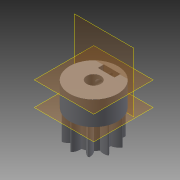
# Autodesk Inventor part: sj-small-gear
Saved by Autodesk Inventor 2014 (Build 180170000, 170)
## iProperties
Created: 2013-11-16
Part Number: sj-small-gear
Material: Generic
Document SubType Name: Modeling
Designer: stephen
Density: 1 g/cm^3
Appearance: Default
Author: stephen
Autodesk Inventor part; units mm, degrees
ref_plane "YZ Plane" through (0, 0, 0) normal (1, 0, 0) x (0, 1, 0)
ref_plane "XZ Plane" through (0, 0, 0) normal (0, 1, 0) x (-1, 0, 0)
ref_plane "XY Plane" through (0, 0, 0) normal (0, 0, 1) x (1, 0, 0)
ref_plane "Work Plane1" through (0, 0, 8) normal (0, 0, 1) x (1, 0, 0)
sketch "Sketch1" plane through (0, 0, 0) normal (0, 0, 1) x (1, 0, 0)
  circle A0 centre (0, 0) radius 2.6023
  line L0 (-0.1767, 8.453) -> (0.1689, 8.453)
  line L1 (0.1689, 8.453) -> (0.9579, 5.5085) construction
  arc A1 (-0.1767, 8.453) -> (-0.9656, 5.5084) centre (2.8217, 6.0717) ccw
  line L2 (-5.1115, 6.7348) -> (-4.8319, 6.9379)
  arc A2 (-2.4629, 5.0195) -> (-4.8319, 6.9379) centre (-5.8579, 3.249) ccw
  line L3 (-4.8319, 6.9379) -> (-2.4629, 5.0195) construction
  arc A3 (-5.1115, 6.7348) -> (-4.0189, 3.8888) centre (-1.286, 6.5706) ccw
  line L4 (-8.0939, 2.4441) -> (-7.9871, 2.7727)
  arc A4 (-4.9429, 2.6132) -> (-7.9871, 2.7727) centre (-6.6488, -0.8147) ccw
  line L5 (-7.9871, 2.7727) -> (-4.9429, 2.6132) construction
  arc A5 (-8.0939, 2.4441) -> (-5.5371, 0.7838) centre (-4.9025, 4.5598) ccw
  line L6 (-7.9847, -2.7801) -> (-8.0915, -2.4515)
  arc A6 (-5.5349, -0.7913) -> (-8.0915, -2.4515) centre (-4.9001, -4.5672) ccw
  line L7 (-8.0915, -2.4515) -> (-5.5349, -0.7913) construction
  arc A7 (-7.9847, -2.7801) -> (-4.9404, -2.6205) centre (-6.6464, 0.8073) ccw
  line L8 (-4.8256, -6.9425) -> (-5.1052, -6.7393)
  arc A8 (-4.0128, -3.8935) -> (-5.1052, -6.7393) centre (-1.2798, -6.5752) ccw
  line L9 (-5.1052, -6.7393) -> (-4.0128, -3.8935) construction
  line L10 (0.1767, -8.453) -> (-0.1689, -8.453)
  arc A9 (-0.9579, -5.5085) -> (-0.1689, -8.453) centre (2.8295, -6.0717) ccw
  line L11 (-0.1689, -8.453) -> (-0.9579, -5.5085) construction
  arc A10 (0.1767, -8.453) -> (0.9656, -5.5084) centre (-2.8217, -6.0717) ccw
  line L12 (5.1115, -6.7348) -> (4.8319, -6.9379)
  arc A11 (2.4629, -5.0195) -> (4.8319, -6.9379) centre (5.8579, -3.249) ccw
  line L13 (4.8319, -6.9379) -> (2.4629, -5.0195) construction
  arc A12 (5.1115, -6.7348) -> (4.0189, -3.8888) centre (1.286, -6.5706) ccw
  line L14 (8.0939, -2.4441) -> (7.9871, -2.7727)
  arc A13 (3.3182, -1.074) -> (8.2332, -2.671) centre (6.6488, 0.8147) ccw
  line L15 (7.9871, -2.7727) -> (4.9429, -2.6132) construction
  line L16 (7.9847, 2.7801) -> (8.0915, 2.4515)
  arc A14 (5.5349, 0.7913) -> (8.0915, 2.4515) centre (4.9001, 4.5672) ccw
  line L17 (8.0915, 2.4515) -> (4.0908, -0.1465) construction
  arc A15 (7.9847, 2.7801) -> (4.9404, 2.6205) centre (6.6464, -0.8073) ccw
  line L18 (4.8256, 6.9425) -> (5.1052, 6.7393)
  arc A16 (4.0128, 3.8935) -> (5.1052, 6.7393) centre (1.2798, 6.5752) ccw
  line L19 (5.1052, 6.7393) -> (4.0128, 3.8935) construction
  arc A17 (-5.5371, 0.7838) -> (-5.536, -0.7919) centre (0, 0) ccw
  arc A18 (-4.0189, 3.8888) -> (-4.9442, 2.6133) centre (0, 0) ccw
  arc A19 (2.4565, 5.0239) -> (0.9575, 5.5098) centre (0, 0) ccw
  arc A20 (4.9404, 2.6205) -> (4.0132, 3.8947) centre (0, 0) ccw
  arc A21 (4.9442, -2.6133) -> (5.536, 0.7919) centre (0, 0) ccw
  arc A22 (2.4639, -5.0203) -> (4.9442, -2.6133) centre (0, 0) ccw
  arc A23 (0.9656, -5.5084) -> (2.4639, -5.0203) centre (0, 0) ccw
  arc A24 (-4.9404, -2.6205) -> (-4.0132, -3.8947) centre (0, 0) ccw
  arc A25 (-2.4565, -5.0239) -> (-0.9575, -5.5098) centre (0, 0) ccw
  arc A26 (0.9579, 5.5085) -> (0.1689, 8.453) centre (-2.8295, 6.0717) ccw
  arc A27 (-2.1474, 2.3039) -> (-1.5764, 2.4536) centre (-2.8295, 6.0717) ccw
  arc A28 (-3.1006, 2.2523) -> (-3.0363, 2.2483) centre (-2.8295, 6.0717) ccw
  arc A29 (4.8256, 6.9425) -> (2.4565, 5.0239) centre (5.8516, 3.2535) ccw
  circle A30 centre (4.9025, -4.5598) radius 3.829
  arc A31 (1.7403, -2.4009) -> (1.7114, -2.4439) centre (4.9025, -4.5598) ccw
  arc A32 (1.1846, -3.6447) -> (1.1248, -3.9359) centre (4.9025, -4.5598) ccw
  arc A33 (-4.8256, -6.9425) -> (-2.4565, -5.0239) centre (-5.8516, -3.2535) ccw
  arc A34 (-2.1424, -2.3034) -> (-2.3452, -1.7153) centre (-5.8516, -3.2535) ccw
  arc A35 (-0.9656, 5.5084) -> (-2.4639, 5.0203) centre (0, 0) ccw
  arc A36 (-4.0189, 3.8888) -> (-4.9442, 2.6133) centre (0, 0) ccw
  point P0 (-0.7682, 6.1639)
  point P1 (0.7605, 6.1646)
  point P2 (-4.2445, 4.5351)
  point P3 (-3.0082, 5.4342)
  point P4 (-6.0996, 1.1741)
  point P5 (-5.6279, 2.6282)
  point P6 (-5.6248, -2.6354)
  point P7 (-6.0979, -1.1817)
  point P8 (-3.0015, -5.4382)
  point P9 (-4.2387, -4.5403)
  point P10 (0.7682, -6.1639)
  point P11 (-0.7605, -6.1646)
  point P12 (4.2445, -4.5351)
  point P13 (3.0082, -5.4342)
  point P14 (6.0996, -1.1741)
  point P15 (5.6279, -2.6282)
  point P16 (5.6248, 2.6354)
  point P17 (6.0979, 1.1817)
  point P18 (3.0015, 5.4382)
  point P19 (4.2387, 4.5403)
  constraints: 81 point on circle, 40 end point, 37 centre point, 15 point on line, 4 coincident, 1 horizontal
sketch "Sketch2" plane through (0, 0, 8) normal (0, 0, 1) x (1, 0, 0)
  circle A0 centre (0, 0) radius 2.6023 projected
  arc A1 (-5.2272, 2.3957) -> (-5.6389, 1.125) centre (0, 0) ccw projected
  circle A2 centre (0, 0) radius 8.8963
  dimension "d8" = 17.7926
  constraints: 1 centre point, 1 coincident
  measures "d8" diameter of A2
extrude "Extrusion2" add sketch "Sketch2" along normal blind 8.85
ref_plane "Work Plane2" through (0, 0, 16.85) normal (0, 0, 1) x (1, 0, 0)
sketch "Sketch3" plane through (0, 0, 16.85) normal (0, 0, 1) x (1, 0, 0)
  circle A0 centre (0, 0) radius 2.6023 projected
  circle A1 centre (0, 0) radius 8.8963 projected
  line L0 (0, 6.8373) -> (3.0745, 6.8373)
  line L1 (3.0745, 6.8373) -> (3.0745, 4.6023)
  line L2 (3.0745, 4.6023) -> (0, 4.6023)
  line L3 (0, 6.8373) -> (-3.0745, 6.8373)
  line L4 (-3.0745, 6.8373) -> (-3.0745, 4.6023)
  line L5 (-3.0745, 4.6023) -> (0, 4.6023)
  line L6 (0, -4.8344) -> (3.0745, -4.8344)
  line L7 (3.0745, -4.8344) -> (3.0745, -7.0696)
  line L8 (3.0745, -7.0696) -> (0, -7.0696)
  line L9 (0, -4.8344) -> (-3.0745, -4.8344)
  line L10 (-3.0745, -4.8344) -> (-3.0745, -7.0696)
  line L11 (-3.0745, -7.0696) -> (0, -7.0696)
  line L12 (0, -9.0696) -> (0, -7.0696)
  line L13 (0, 2.6023) -> (0, 3.7788)
  line L14 (0, 3.7788) -> (0, 4.6023)
  dimension "d10" = 2.235
  dimension "d11" = 2
  dimension "d31" = 2.2352
  dimension "d32" = 6.149
  dimension "d33" = 6.149
  constraints: 30 end point, 3 collinear, 3 perpendicular, 2 horizontal, 2 parallel, 1 vertical, 1 vertical alignment, 1 other
  measures "d10" distance of L0.end L1.end
  measures "d31" distance of L6.end L7.end
  measures "d32" distance between parallel lines of L10 L7
  measures "d33" distance between parallel lines of L4 L1
extrude "Extrusion3" cut sketch "Sketch3" against normal blind 8 contours L5 L4 L3 L0 L1 L2
ref_plane "Work Plane3" through (-2.75, 6.6023, 16.85) normal (0, -1, 0) x (1, 0, 0)
sketch "Sketch4" plane through (-2.75, 6.6023, 16.85) normal (0, -1, 0) x (1, 0, 0)
  line L0 (5.5, 0) -> (5.5, -8) projected
  line L1 (2.75, 0.553) -> (2.75, -3.197)
  circle A0 centre (2.75, -2.8775) radius 1.75
  point P0 (2.75, -16.85)
  dimension "d14" = 3.75
  dimension "d15" = 3.5
  constraints: 2 end point, 1 centre point, 1 parallel, 1 point on line
  measures "d14" distance of L1.start L1.end
  measures "d15" diameter of A0
extrude "Extrusion4" cut sketch "Sketch4" along normal mid plane 9
sketch "Sketch5" plane through (0, 0, 8) normal (0, 0, -1) x (-1, 0, 0)
  circle A0 centre (0, 0) radius 2.6023 projected
  circle A1 centre (0, 0) radius 8.8963 projected
  line L0 (-0.1767, 8.453) -> (0.169, 8.453)
  line L1 (0.1689, 8.453) -> (0.9579, 5.5085) construction
  arc A2 (0.9579, 5.5085) -> (0.1689, 8.453) centre (-2.8295, 6.0717) ccw
  circle A3 centre (0, 0) radius 2.6023
  arc A4 (-0.1767, 8.453) -> (-0.9656, 5.5085) centre (2.8217, 6.0717) ccw
  arc A5 (0.9575, 5.5099) -> (0.169, 8.453) centre (-2.8254, 6.0736) ccw
  line L2 (0.1689, 8.453) -> (-0.1767, 8.453)
  arc A6 (-0.1767, 8.453) -> (-0.9656, 5.5085) centre (2.8217, 6.0717) ccw
  line L3 (-5.1115, 6.7348) -> (-4.8318, 6.9379)
  line L4 (-4.8319, 6.9379) -> (-2.4629, 5.0195) construction
  arc A7 (-2.4629, 5.0195) -> (-4.8319, 6.9379) centre (-5.8579, 3.249) ccw
  arc A8 (-5.1115, 6.7348) -> (-4.019, 3.8889) centre (-1.286, 6.5706) ccw
  arc A9 (-2.464, 5.0204) -> (-4.8318, 6.9379) centre (-5.8558, 3.2529) ccw
  line L5 (-4.8319, 6.9379) -> (-5.1115, 6.7348)
  arc A10 (-5.1115, 6.7348) -> (-4.019, 3.8889) centre (-1.286, 6.5706) ccw
  line L6 (-8.0939, 2.4441) -> (-7.987, 2.7728)
  line L7 (-7.9871, 2.7727) -> (-4.9429, 2.6132) construction
  arc A11 (-4.9429, 2.6132) -> (-7.9871, 2.7727) centre (-6.6488, -0.8147) ccw
  arc A12 (-8.0939, 2.4441) -> (-5.5373, 0.7839) centre (-4.9025, 4.5598) ccw
  arc A13 (-4.9444, 2.6133) -> (-7.987, 2.7728) centre (-6.6494, -0.8103) ccw
  line L8 (-7.9871, 2.7727) -> (-8.0939, 2.4441)
  arc A14 (-8.0939, 2.4441) -> (-5.5373, 0.7839) centre (-4.9025, 4.5598) ccw
  line L9 (-7.9847, -2.7801) -> (-8.0915, -2.4514)
  line L10 (-8.0915, -2.4515) -> (-5.5349, -0.7913) construction
  arc A15 (-5.5349, -0.7913) -> (-8.0915, -2.4515) centre (-4.9001, -4.5672) ccw
  arc A16 (-7.9847, -2.7801) -> (-4.9405, -2.6206) centre (-6.6464, 0.8073) ccw
  arc A17 (-5.5361, -0.792) -> (-8.0915, -2.4514) centre (-4.9032, -4.564) ccw
  line L11 (-8.0915, -2.4515) -> (-7.9847, -2.7801)
  arc A18 (-7.9847, -2.7801) -> (-4.9405, -2.6206) centre (-6.6464, 0.8073) ccw
  line L12 (-4.8256, -6.9425) -> (-5.1053, -6.7393)
  line L13 (-5.1052, -6.7393) -> (-4.0128, -3.8935) construction
  arc A19 (-4.0128, -3.8935) -> (-5.1052, -6.7393) centre (-1.2798, -6.5752) ccw
  arc A20 (-4.8256, -6.9425) -> (-2.4566, -5.0241) centre (-5.8516, -3.2535) ccw
  arc A21 (-4.0133, -3.8948) -> (-5.1053, -6.7393) centre (-1.2842, -6.5744) ccw
  line L14 (-5.1052, -6.7393) -> (-4.8256, -6.9425)
  arc A22 (-4.8256, -6.9425) -> (-2.4566, -5.0241) centre (-5.8516, -3.2535) ccw
  line L15 (0.1767, -8.453) -> (-0.169, -8.453)
  line L16 (-0.1689, -8.453) -> (-0.9579, -5.5085) construction
  arc A23 (-0.9579, -5.5085) -> (-0.1689, -8.453) centre (2.8295, -6.0717) ccw
  arc A24 (0.1767, -8.453) -> (0.9656, -5.5085) centre (-2.8217, -6.0717) ccw
  arc A25 (-0.9575, -5.5099) -> (-0.169, -8.453) centre (2.8254, -6.0736) ccw
  line L17 (-0.1689, -8.453) -> (0.1767, -8.453)
  arc A26 (0.1767, -8.453) -> (0.9656, -5.5085) centre (-2.8217, -6.0717) ccw
  line L18 (5.1115, -6.7348) -> (4.8318, -6.9379)
  line L19 (4.8319, -6.9379) -> (2.4629, -5.0195) construction
  arc A27 (2.4629, -5.0195) -> (4.8319, -6.9379) centre (5.8579, -3.249) ccw
  arc A28 (5.1115, -6.7348) -> (4.019, -3.8889) centre (1.286, -6.5706) ccw
  arc A29 (2.464, -5.0204) -> (4.8318, -6.9379) centre (5.8558, -3.2529) ccw
  line L20 (4.8319, -6.9379) -> (5.1115, -6.7348)
  arc A30 (5.1115, -6.7348) -> (4.019, -3.8889) centre (1.286, -6.5706) ccw
  line L21 (8.0939, -2.4441) -> (7.987, -2.7728)
  line L22 (7.9871, -2.7727) -> (4.9429, -2.6132) construction
  arc A31 (4.9429, -2.6132) -> (7.9871, -2.7727) centre (6.6488, 0.8147) ccw
  arc A32 (8.0939, -2.4441) -> (5.5373, -0.7839) centre (4.9025, -4.5598) ccw
  arc A33 (4.9444, -2.6133) -> (7.987, -2.7728) centre (6.6494, 0.8103) ccw
  line L23 (7.9871, -2.7727) -> (8.0939, -2.4441)
  arc A34 (8.0939, -2.4441) -> (5.5373, -0.7839) centre (4.9025, -4.5598) ccw
  line L24 (7.9847, 2.7801) -> (8.0915, 2.4514)
  line L25 (8.0915, 2.4515) -> (5.5349, 0.7913) construction
  arc A35 (5.5349, 0.7913) -> (8.0915, 2.4515) centre (4.9001, 4.5672) ccw
  arc A36 (7.9847, 2.7801) -> (4.9405, 2.6206) centre (6.6464, -0.8073) ccw
  arc A37 (5.5361, 0.792) -> (8.0915, 2.4514) centre (4.9032, 4.564) ccw
  line L26 (8.0915, 2.4515) -> (7.9847, 2.7801)
  arc A38 (7.9847, 2.7801) -> (4.9405, 2.6206) centre (6.6464, -0.8073) ccw
  line L27 (4.8256, 6.9425) -> (5.1053, 6.7393)
  line L28 (5.1052, 6.7393) -> (4.0128, 3.8935) construction
  arc A39 (4.0128, 3.8935) -> (5.1052, 6.7393) centre (1.2798, 6.5752) ccw
  arc A40 (4.8256, 6.9425) -> (2.4566, 5.0241) centre (5.8516, 3.2535) ccw
  arc A41 (4.0133, 3.8948) -> (5.1053, 6.7393) centre (1.2842, 6.5744) ccw
  line L29 (5.1052, 6.7393) -> (4.8256, 6.9425)
  arc A42 (4.8256, 6.9425) -> (2.4566, 5.0241) centre (5.8516, 3.2535) ccw
  arc A43 (2.4566, 5.0241) -> (0.9575, 5.5099) centre (0, 0) ccw
  arc A44 (4.9405, 2.6206) -> (4.0133, 3.8948) centre (0, 0) ccw
  arc A45 (5.5373, -0.7839) -> (5.5361, 0.792) centre (0, 0) ccw
  arc A46 (4.019, -3.8889) -> (4.9444, -2.6133) centre (0, 0) ccw
  arc A47 (0.9656, -5.5085) -> (2.464, -5.0204) centre (0, 0) ccw
  arc A48 (-2.4566, -5.0241) -> (-0.9575, -5.5099) centre (0, 0) ccw
  arc A49 (-4.9405, -2.6206) -> (-4.0133, -3.8948) centre (0, 0) ccw
  arc A50 (-5.5373, 0.7839) -> (-5.5361, -0.792) centre (0, 0) ccw
  arc A51 (-0.9656, 5.5085) -> (-2.464, 5.0204) centre (0, 0) ccw
  arc A52 (-4.019, 3.8889) -> (-4.9444, 2.6133) centre (0, 0) ccw
  point P0 (-0.7682, 6.1639)
  point P1 (0.7605, 6.1646)
  point P2 (-1.286, 6.5706)
  point P3 (1.2798, 6.5752)
  point P4 (0.9575, 5.5098)
  point P5 (-4.9025, 4.5598)
  point P6 (-4.2445, 4.5351)
  point P7 (-2.4639, 5.0203)
  point P8 (-3.0082, 5.4342)
  point P9 (-2.8295, 6.0717)
  point P10 (-6.6464, 0.8073)
  point P11 (-6.0996, 1.1741)
  point P12 (-4.9442, 2.6133)
  point P13 (-5.6279, 2.6282)
  point P14 (-5.8579, 3.249)
  point P15 (-5.8516, -3.2535)
  point P16 (-5.6248, -2.6354)
  point P17 (-5.536, -0.7919)
  point P18 (-6.0979, -1.1817)
  point P19 (-6.6488, -0.8147)
  point P20 (-2.8217, -6.0717)
  point P21 (-3.0015, -5.4382)
  point P22 (-4.0132, -3.8947)
  point P23 (-4.2387, -4.5403)
  point P24 (-4.9001, -4.5672)
  point P25 (1.286, -6.5706)
  point P26 (0.7682, -6.1639)
  point P27 (-0.9575, -5.5098)
  point P28 (-0.7605, -6.1646)
  point P29 (-1.2798, -6.5752)
  point P30 (4.9025, -4.5598)
  point P31 (4.2445, -4.5351)
  point P32 (2.4639, -5.0203)
  point P33 (3.0082, -5.4342)
  point P34 (2.8295, -6.0717)
  point P35 (6.6464, -0.8073)
  point P36 (6.0996, -1.1741)
  point P37 (4.9442, -2.6133)
  point P38 (5.6279, -2.6282)
  point P39 (5.8579, -3.249)
  point P40 (5.8516, 3.2535)
  point P41 (5.6248, 2.6354)
  point P42 (5.536, 0.7919)
  point P43 (6.0979, 1.1817)
  point P44 (6.6488, 0.8147)
  point P45 (2.8217, 6.0717)
  point P46 (3.0015, 5.4382)
  point P47 (4.0132, 3.8947)
  point P48 (4.2387, 4.5403)
  point P49 (4.9001, 4.5672)
  dimension "d27" = 360
  constraints: 100 point on circle, 60 end point, 51 centre point, 30 point on line, 2 coincident, 1 concentric, 1 horizontal, 221 other
extrude "Extrusion5" add sketch "Sketch5" along normal blind 10 contours L0 A2 A43 A40 L27 A39 A44 A36 L24 A35 A45 A32 L21 A31 A46 A28 L18 A27 A47 A24 L15 A23 A48 A20 L12 A19 A49 A16 L9 A15 A50 A12 L6 A11 A52 A8 L3 A7 A51 A4
body "Solid1"
